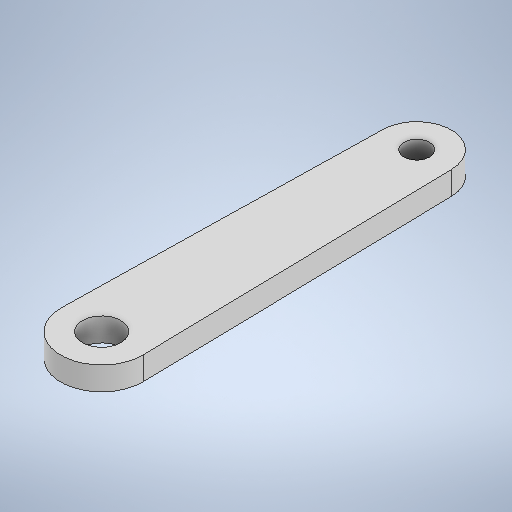
# Autodesk Inventor part: servo_leg
Saved by Autodesk Inventor 2025.2 (Build 292293000, 293)
## iProperties
Created: 2025-02-03
Part Number: servo_leg
Material: Типовые
Document SubType Name: Modeling
Designer: ignat
Density: 1 g/cm^3
Appearance: По умолчанию
Author: ignat
Autodesk Inventor part; units mm, degrees
ref_plane "YZ Plane" through (0, 0, 0) normal (1, 0, 0) x (0, 1, 0)
ref_plane "XZ Plane" through (0, 0, 0) normal (0, 1, 0) x (-1, 0, 0)
ref_plane "XY Plane" through (0, 0, 0) normal (0, 0, 1) x (1, 0, 0)
sketch "Эскиз1" plane through (0, 0, 0) normal (0, 1, 0) x (-1, 0, 0)
  line L0 (0, 17) -> (0, 17)
  line L1 (0, -17) -> (0, -17)
  arc A0 (3.4993, 13.4287) -> (0, 17) centre (0, 13.5) ccw
  circle A1 centre (0, 13.5) radius 1.65
  circle A2 centre (0, -13.5) radius 1.1
  line L2 (3.4993, 13.4287) -> (2.9494, -13.5601)
  arc A3 (0, -16.45) -> (2.9494, -13.5601) centre (0, -13.5) ccw
  arc A4 (0, 17) -> (-3.4993, 13.4287) centre (0, 13.5) ccw
  line L3 (-3.4993, 13.4287) -> (-2.9494, -13.5601)
  arc A5 (-2.9494, -13.5601) -> (0, -16.45) centre (0, -13.5) ccw
  point P0 (0, 0)
  dimension "d2" = 3.5
  dimension "d4" = 2.2
  dimension "d5" = 3.3
  constraints: 8 end point, 8 point on circle, 6 centre point, 2 tangent, 1 coincident, 1 horizontal, 1 parallel
  measures "d2" radius of A0
  measures "d4" diameter of A2
  measures "d5" diameter of A1
extrude "Выдавливание1" add sketch "Эскиз1" along normal blind 2
